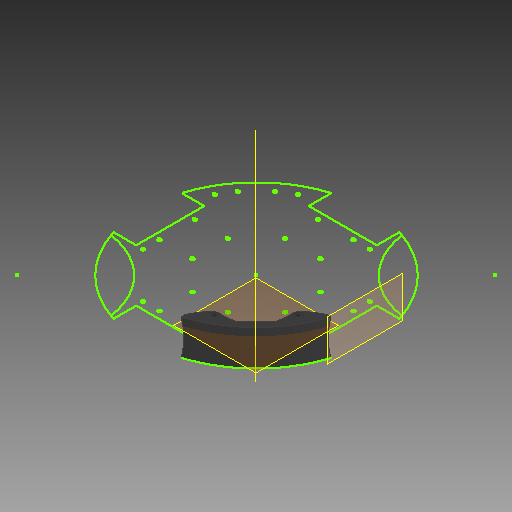
# Autodesk Inventor part: protect
Saved by Autodesk Inventor 2020 (Build 240168000, 168)
## iProperties
Created: 2024-09-14
Part Number: protect
Material: Типовые
Document SubType Name: Modeling
Designer: Ivan
Density: 1 g/cm^3
Appearance: Черный — литой
Author: Ivan
Autodesk Inventor part; units mm, degrees
ref_plane "YZ Plane" through (0, 0, 0) normal (1, 0, 0) x (0, 1, 0)
ref_plane "XZ Plane" through (0, 0, 0) normal (0, 1, 0) x (-1, 0, 0)
ref_plane "XY Plane" through (0, 0, 0) normal (0, 0, 1) x (1, 0, 0)
sketch "Эскиз1" plane through (0, 0, 0) normal (0, 1, 0) x (-1, 0, 0)
  arc A0 (-31, 99.2724) -> (-99.2724, 31) centre (0, 0) ccw
  circle A1 centre (-74.5664, 57.67) radius 1.5
  circle A2 centre (-82.9015, 44.87) radius 1.5
  circle A3 centre (-57.67, 74.5664) radius 1.5
  circle A4 centre (-44.87, 82.9015) radius 1.5
  line L0 (-31, 99.2724) -> (-31, 78.7724)
  line L1 (-31, 78.7724) -> (31, 78.7724)
  circle A5 centre (-16, 72.43) radius 1.5
  circle A6 centre (16, 72.43) radius 1.5
  circle A7 centre (31, 72.43) radius 1.5
  line L2 (31, 78.7724) -> (31, 99.2724)
  circle A8 centre (16, 42.22) radius 1.5
  circle A9 centre (-16, 42.22) radius 1.5
  circle A10 centre (-42.22, 16) radius 1.5
  circle A11 centre (-72.43, 16) radius 1.5
  line L3 (-99.2724, 31) -> (-78.7724, 31)
  line L4 (-78.7724, 31) -> (-78.7724, -31)
  arc A12 (34.57, 98.0863) -> (98.0863, 34.57) centre (109.0212, 109.0212) ccw
  circle A13 centre (72.43, 31) radius 1.5
  line L5 (99.2724, 31) -> (78.7724, 31)
  line L6 (78.7724, 31) -> (78.7724, -31)
  circle A14 centre (72.43, 16) radius 1.5
  circle A15 centre (42.22, 16) radius 1.5
  circle A16 centre (42.22, -16) radius 1.5
  circle A17 centre (72.43, -16) radius 1.5
  circle A18 centre (82.9015, -44.87) radius 1.5
  line L7 (78.7724, -31) -> (99.2724, -31)
  arc A19 (31, -99.2724) -> (99.2724, -31) centre (0, 0) ccw
  circle A20 centre (74.5664, -57.67) radius 1.5
  circle A21 centre (16, -42.22) radius 1.5
  circle A22 centre (57.67, -74.5664) radius 1.5
  circle A23 centre (44.87, -82.9015) radius 1.5
  circle A24 centre (16, -72.43) radius 1.5
  line L8 (31, -78.7724) -> (31, -99.2724)
  line L9 (-31, -78.7724) -> (31, -78.7724)
  circle A25 centre (-16, -72.43) radius 1.5
  circle A26 centre (-16, -42.22) radius 1.5
  circle A27 centre (-31, -72.43) radius 1.5
  circle A28 centre (-42.22, -16) radius 1.5
  circle A29 centre (-72.43, -16) radius 1.5
  circle A30 centre (-72.43, -31) radius 1.5
  line L10 (-78.7724, -31) -> (-99.2724, -31)
  line L11 (-31, -99.2724) -> (-31, -78.7724)
  arc A31 (-34.57, -98.0863) -> (-31, -99.2724) centre (0, 0) ccw
  arc A32 (-99.2724, -31) -> (-98.0863, -34.57) centre (0, 0) ccw
  arc A33 (-34.57, -98.0863) -> (-98.0863, -34.57) centre (-109.0212, -109.0212) ccw
  line L12 (-73.5391, 73.5391) -> (73.5391, -73.5391) construction
  arc A34 (34.57, 98.0863) -> (31, 99.2724) centre (0, 0) ccw
  arc A35 (99.2724, 31) -> (98.0863, 34.57) centre (0, 0) ccw
  arc A36 (-98.0863, -34.57) -> (-34.57, -98.0863) centre (0, 0) ccw
  arc A37 (98.0863, 34.57) -> (34.57, 98.0863) centre (0, 0) ccw
  constraints: 38 centre point, 26 end point, 23 point on circle, 5 coincident, 1 horizontal, 1 perpendicular, 1 symmetric about line, 2 other
sketch "Эскиз2" plane through (0, 0, 0) normal (0, 1, 0) x (-1, 0, 0)
  circle A0 centre (-82.9015, 44.87) radius 1.5 projected
  circle A1 centre (-44.87, 82.9015) radius 1.5 projected
  circle A2 centre (-44.87, 82.9015) radius 2
  circle A3 centre (-82.9015, 44.87) radius 2
  arc A4 (-31, 99.2724) -> (-99.2724, 31) centre (0, 0) ccw projected
  arc A5 (-31, 99.2724) -> (-99.2724, 31) centre (0, 0) ccw
  circle A6 centre (-44.87, 82.9015) radius 4
  circle A7 centre (-82.9015, 44.87) radius 4
  line L0 (-73.5391, 73.5391) -> (73.5391, -73.5391) construction
  line L1 (-31, 99.2724) -> (-31, 78.7724) projected
  line L2 (-99.2724, 31) -> (-78.7724, 31) projected
  arc A8 (-31, 95.7724) -> (-95.7724, 31) centre (0, 0) ccw construction
  line L3 (-31, 95.7724) -> (-95.7724, 31) construction
  line L4 (-42.0416, 85.7299) -> (-47.6984, 80.0731) construction
  circle A9 centre (-57.67, 74.5664) radius 1.5 construction
  circle A10 centre (-74.5664, 57.67) radius 1.5 construction
  circle A11 centre (-57.67, 74.5664) radius 3.5
  circle A12 centre (-74.5664, 57.67) radius 3.5
  line L5 (-60.1449, 77.0413) -> (-55.1951, 72.0915) construction
  line L6 (-77.0413, 60.1449) -> (-72.0915, 55.1951) construction
  line L7 (-60.1449, 77.0413) -> (-77.0413, 60.1449)
  line L8 (-44.87, 82.9015) -> (-42.0416, 80.0731) construction
  arc A13 (-42.0416, 80.0731) -> (-31, 95.7724) centre (-70.386, 111.7408) ccw
  line L9 (-42.0416, 80.0731) -> (-47.6984, 80.0731) construction
  line L10 (-44.87, 82.9015) -> (-44.87, 78.9015) construction
  line L11 (-55.1951, 77.0413) -> (-60.1449, 72.0915) construction
  line L12 (-60.1449, 77.0413) -> (-55.1951, 77.0413) construction
  line L13 (-57.67, 74.5664) -> (-57.67, 78.0664) construction
  arc A14 (-44.87, 78.9015) -> (-57.67, 78.0664) centre (-48.6366, 38.1205) ccw
  arc A15 (-78.0664, 57.67) -> (-78.9015, 44.87) centre (-38.1205, 48.6366) ccw
  line L14 (-82.9015, 44.87) -> (-80.0731, 42.0416) construction
  arc A16 (-95.7724, 31) -> (-80.0731, 42.0416) centre (-111.7408, 70.386) ccw
  point P0 (-95.7724, 31)
  point P1 (-95.7724, 31)
  point P2 (-78.9015, 44.87)
  dimension "d3" = 8
  dimension "d0" = 4
  dimension "d1" = 4
  dimension "d2" = 8
  dimension "d4" = 3.5
  dimension "d5" = 3.5
  dimension "d7" = 7
  dimension "d8" = 7
  dimension "d9" = 42.5
  constraints: 24 end point, 24 point on circle, 11 centre point, 7 coincident, 5 midpoint, 4 parallel, 3 symmetric about line, 2 horizontal, 2 perpendicular, 2 point on line, 1 concentric, 1 equal radius, 4 other
  measures "d0" diameter of A2
  measures "d1" diameter of A3
  measures "d2" diameter of A6
  measures "d4" distance of L3.start L1.start
  measures "d5" distance of point (-95.772, 31) L2.start
  measures "d7" diameter of A11
  measures "d8" diameter of A12
  measures "d9" radius of A13
extrude "Выдавливание1" add sketch "Эскиз2" along normal blind 32 contours L1 A13 A6 A14 A11 L7 A12 A15 A7 A16 L2 A4 | A6 A14 | A7 A15 picked at (-41.5746, 83.2174) picked at (-80.8909, 42.2371)
ref_plane "РабПлоскость1" through (0, 25.3, 0) normal (0, 1, 0) x (1, 0, 0)
sketch "Эскиз3" plane through (0, 25.3, 0) normal (0, 1, 0) x (1, 0, 0)
  circle A0 centre (44.87, -82.9015) radius 2 projected
  circle A1 centre (82.9015, -44.87) radius 2 projected
  point P0 (0, 0)
extrude "Выдавливание2" add sketch "Эскиз3" against normal blind 20.6
ref_plane "РабПлоскость2" through (99.2724, 32, 31) normal (1, 0, 0) x (0, -1, 0)
sketch "Эскиз4" plane through (99.2724, 32, 31) normal (1, 0, 0) x (0, -1, 0)
  arc A0 (0, 0) -> (32, 0) centre (16, 72.5568) ccw
  line L0 (32, 0) -> (0, 0) projected
  line L1 (0, 0) -> (32, 0)
  point P0 (32, 31)
  dimension "d15" = 74.3
  constraints: 2 coincident, 2 end point, 2 point on circle, 1 centre point, 1 horizontal
  measures "d15" radius of A0
extrude "Выдавливание3" cut sketch "Эскиз4" against normal blind 20.6
ref_plane "РабПлоскость3" through (73.5391, 32, 73.5391) normal (0.7071068, 0, -0.7071068) x (0, -1, 0)
mirror "Зеркальное отражение1" about plane through (73.5391, 32, 73.5391) normal (0.7071068, 0, -0.7071068) of "Выдавливание3"
equation "\"d5\" = d4"
